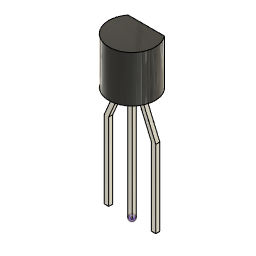
3D Model (Autodesk Fusion 360 design; units mm, degrees)
Autodesk Fusion 360 part; units mm, degrees
sketch "Sketch1" plane through (0, 0, 0) normal (0, 0, 1) x (1, 0, 0)
  circle A0 centre (0, 0) radius 2.6
  line L0 (0.25, 0.2248) -> (-0.25, 0.2248)
  line L1 (-0.25, 0.2248) -> (-0.25, -0.2248)
  line L2 (-0.25, -0.2248) -> (0.25, -0.2248)
  line L3 (0.25, -0.2248) -> (0.25, 0.2248)
  line L4 (0.25, 0.2248) -> (-0.25, -0.2248) construction
  line L5 (-0.25, 0.2248) -> (0.25, -0.2248) construction
  line L6 (-1, -0.2236) -> (-1.5, -0.2236)
  line L7 (-1.5, -0.2236) -> (-1.5, 0.2262)
  line L8 (-1.5, 0.2262) -> (-1, 0.2262)
  line L9 (-1, 0.2262) -> (-1, -0.2236)
  line L10 (-1, -0.2236) -> (-1.5, 0.2262) construction
  line L11 (-1.5, -0.2236) -> (-1, 0.2262) construction
  line L12 (1.5, -0.2247) -> (1, -0.2247)
  line L13 (1, -0.2247) -> (1, 0.225)
  line L14 (1, 0.225) -> (1.5, 0.225)
  line L15 (1.5, 0.225) -> (1.5, -0.2247)
  line L16 (1.5, -0.2247) -> (1, 0.225) construction
  line L17 (1, -0.2247) -> (1.5, 0.225) construction
  point P0 (-1.25, 0.0013)
  point P1 (1.25, 0.0002)
  dimension "d7" = 0.5
  dimension "d9" = 0.5
  dimension "d10" = 0.5
  constraint coincident A0.centre origin
  constraint horizontal L0
  constraint perpendicular L0 L1
  constraint parallel L0 L2
  constraint parallel L1 L3
  constraint coincident L4 A0.centre
  constraint coincident L5 A0.centre
  constraint horizontal L6
  constraint perpendicular L6 L7
  constraint parallel L6 L8
  constraint parallel L7 L9
  constraint coincident L10 P0
  constraint coincident L11 P0
  constraint horizontal L12
  constraint perpendicular L12 L13
  constraint parallel L12 L14
  constraint parallel L13 L15
  constraint coincident L16 P1
  constraint coincident L17 P1
  measures "d7" distance of L1.end L2.end
  measures "d9" distance of L7.end L8.end
  measures "d10" distance of L13.end L14.end
extrude "Extrude1" add sketch "Sketch1" along normal blind 5.2
sketch "Sketch2" plane through (0, 0, 0) normal (0, 0, 1) x (1, 0, 0)
sketch "Sketch3" plane through (0, 0, 5.2) normal (0, 0, 1) x (-1, 0, 0)
  line L0 (1.5, -0.2262) -> (1, -0.2262)
  line L1 (1, -0.2262) -> (1, 0.2236)
  line L2 (1, 0.2236) -> (1.5, 0.2236)
  line L3 (1.5, 0.2236) -> (1.5, -0.2262)
  line L4 (-0.25, -0.2248) -> (-0.25, 0.2248)
  line L5 (-0.25, 0.2248) -> (0.25, 0.2248)
  line L6 (0.25, 0.2248) -> (0.25, -0.2248)
  line L7 (0.25, -0.2248) -> (-0.25, -0.2248)
  line L8 (-1, -0.225) -> (-1.5, -0.225)
  line L9 (-1.5, -0.225) -> (-1.5, 0.2247)
  line L10 (-1.5, 0.2247) -> (-1, 0.2247)
  line L11 (-1, 0.2247) -> (-1, -0.225)
  circle A0 centre (0, 0) radius 2.6
  line L12 (-3.3, -1.6) -> (3.3, -1.6)
  line L13 (3.3, -1.6) -> (3.3, -3.6)
  line L14 (3.3, -3.6) -> (-3.3, -3.6)
  line L15 (-3.3, -3.6) -> (-3.3, -1.6)
  line L16 (-3.3, -1.6) -> (3.3, -3.6) construction
  line L17 (3.3, -1.6) -> (-3.3, -3.6) construction
  point P0 (0, -2.6)
  constraint horizontal L12
  constraint perpendicular L12 L13
  constraint parallel L12 L14
  constraint parallel L13 L15
  constraint coincident L16 P0
  constraint coincident L17 P0
  constraint coincident A0 P0
sketch "Sketch7" plane through (0, 0, 0) normal (1, 0, 0) x (0, 1, 0)
extrude "Extrude2" cut sketch "Sketch3" against normal blind 8.6 contours A0 L12 | A0 L12 L13 L14 L15 picked at (-0.6022, -1.6899)
extrude "Extrude3" cut 1 faces at (1.3333, -0.2247, 1.7333) along direction (0, 1, 0) blind 0.5
extrude "Extrude4" add 1 faces at (1.5, -0.058, 1.7333) along direction (-1, 0, 0) blind 0.5
extrude "Extrude5" add 1 faces at (0.25, -0.0749, 1.7333) along direction (-1, 0, 0) blind 0.5
extrude "Extrude6" add 1 faces at (-1, 0.0763, 1.7333) along direction (-1, 0, 0) blind 0.5
move_body "Move1" bodies 1 to x (1, 0, 0) y (0, 1, 0) z (0, 0, 1) at (0, 0, 12.7)
extrude "Extrude12" add sketch "Sketch1" along normal blind 12.7 contours L12 L13 L14 L15
extrude "Extrude14" add sketch "Sketch1" along normal blind 12.7 contours L0 L1 L2 L3
extrude "Extrude15" add sketch "Sketch1" along normal blind 12.7 contours L6 L7 L8 L9
extrude "Extrude16" cut 1 faces at (1.3333, -0.0748, 0) along direction (0, 0, 1) blind 12
sketch "Sketch11" plane through (0, 0, 12) normal (0, 0, -1) x (1, 0, 0)
  line L0 (1, -0.225) -> (1.5, -0.225)
  line L1 (1.5, -0.225) -> (1.5, 0.2247)
  line L2 (1.5, 0.2247) -> (1, 0.2247)
  line L3 (1, 0.2247) -> (1, -0.225)
sketch "Sketch12" plane through (0, 0, 0) normal (0, 1, 0) x (1, 0, 0)
sketch "Sketch15" plane through (0, 0, 0) normal (0, 0, 1) x (1, 0, 0)
  line L0 (2.9002, 0.225) -> (2.3998, 0.225)
  line L1 (2.3998, 0.225) -> (2.3998, -0.225)
  line L2 (2.3998, -0.225) -> (2.9002, -0.225)
  line L3 (2.9002, -0.225) -> (2.9002, 0.225)
  line L4 (2.9002, 0.225) -> (2.3998, -0.225) construction
  line L5 (2.3998, 0.225) -> (2.9002, -0.225) construction
  point P0 (2.65, 0)
  dimension "d66" = 0.45
  constraint horizontal L0
  constraint perpendicular L0 L1
  constraint parallel L0 L2
  constraint parallel L1 L3
  constraint coincident L4 P0
  constraint coincident L5 P0
  measures "d66" distance of L0.end L1.end
sketch "Sketch17" plane through (0, 0.225, 0) normal (0, 1, 0) x (-1, 0, 0)
  line L0 (-1.5, 12) -> (-1, 12)
  line L1 (-1, 12) -> (-1, 12.7)
  line L2 (-1, 12.7) -> (-1.5, 12.7)
  line L3 (-1.5, 12.7) -> (-1.5, 12)
  line L4 (-1.5, 12) -> (-2.9, 8.7)
  constraint coincident L0.start L3.end
sweep "Sweep2" add profiles "Sketch11" path "Sketch17" along L4 section 1
extrude "Extrude18" add 1 faces at (2.5667, -0.0748, 8.7) along direction (0, 0, -1) blind 8.7
extrude "Extrude19" cut 1 faces at (-1.3333, 0.0763, 0) along direction (0, 0, 1) blind 12
sketch "Sketch18" plane through (0, 0, 12) normal (0, 0, -1) x (1, 0, 0)
  line L0 (-1.5, -0.2262) -> (-1, -0.2262)
  line L1 (-1, -0.2262) -> (-1, 0.2236)
  line L2 (-1, 0.2236) -> (-1.5, 0.2236)
  line L3 (-1.5, 0.2236) -> (-1.5, -0.2262)
sketch "Sketch19" plane through (0, 0.2262, 0) normal (0, 1, 0) x (-1, 0, 0)
  line L0 (1, 12) -> (1.5, 12)
  line L1 (1.5, 12) -> (1.5, 12.7)
  line L2 (1.5, 12.7) -> (1, 12.7)
  line L3 (1, 12.7) -> (1, 12)
  line L4 (1.5, 12) -> (2.9, 8.7)
  constraint coincident L0.end L1.start
sweep "Sweep3" add profiles "Sketch18" path "Sketch19" along L4 section 1
extrude "Extrude21" add 1 faces at (-2.5667, 0.0763, 8.7) along direction (0, 0, -1) blind 8.7
sketch "Sketch20" plane through (0, 1.6, 0) normal (0, 1, 0) x (-1, 0, 0)
  line L0 (2.0494, 12.7) -> (2.0494, 17.9)
  line L1 (2.0494, 17.9) -> (-2.0494, 17.9)
  line L2 (-2.0494, 17.9) -> (-2.0494, 12.7)
  line L3 (-2.0494, 12.7) -> (2.0494, 12.7)
  line L4 (-2.0494, 12.7) -> (2.0494, 12.7) construction
  line L5 (2.0494, 12.7) -> (2.0494, 17.9) construction
  line L6 (2.0494, 17.9) -> (-2.0494, 17.9) construction
  line L7 (-2.0494, 17.9) -> (-2.0494, 12.7) construction
  dimension "d89" = 0.4
  text T0 "KSA539CYTA" font "Arial" height 0.4 align centre middle in box 4.0988 x 5.2 at (-2.0494, 12.7) x (1, 0) y (0, 1) spacing 1 kerned
  constraint coincident L0.start
  constraint coincident L1.end
emboss "Emboss4" depth 0.1 profiles "Sketch20" section 1 text T0 onto face at (0.6831, 1.6, 16.1667)
